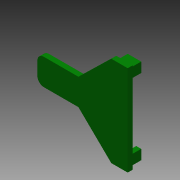
# Autodesk Inventor part: Front Sensor Holder
Saved by Autodesk Inventor 2014 (Build 180170000, 170)
## iProperties
Created: 2016-02-03
Part Number: Front Sensor Holder
Material: Generic
Document SubType Name: Modeling
Designer: Paul
Density: 1 g/cm^3
Appearance: Dark Green
Author: Paul
Autodesk Inventor part; units mm, degrees
ref_plane "YZ Plane" through (0, 0, 0) normal (1, 0, 0) x (0, 1, 0)
ref_plane "XZ Plane" through (0, 0, 0) normal (0, 1, 0) x (-1, 0, 0)
ref_plane "XY Plane" through (0, 0, 0) normal (0, 0, 1) x (1, 0, 0)
sketch "Sketch1" plane through (0, 0, 0) normal (0, 1, 0) x (-1, 0, 0)
  line L0 (6, 8) -> (-15, 8)
  line L1 (-15, -8) -> (6, -8)
  line L2 (10, -4) -> (10, 4)
  line L3 (-45, 0) -> (10, 0) construction
  arc A0 (10, 4) -> (6, 8) centre (6, 4) ccw
  arc A1 (6, -8) -> (10, -4) centre (6, -4) ccw
  line L4 (-35, 27.5) -> (-15, 8)
  line L5 (-15, -8) -> (-35, -27.5)
  line L6 (-35, 27.5) -> (-45, 27.5)
  line L7 (-45, 27.5) -> (-45, -27.5)
  line L8 (-45, -27.5) -> (-35, -27.5)
  point P0 (0, 0)
  point P1 (10, 8)
  point P2 (10, -8)
  dimension "d1" = 16
  dimension "d3" = 10
  dimension "d4" = 4
  dimension "d16" = 20
  dimension "d17" = 10
  dimension "d18" = 55
  dimension "d26" = 25
  constraints: 18 end point, 5 point on line, 4 point on circle, 4 tangent, 3 parallel, 2 centre point, 2 midpoint, 2 vertical, 1 equal length, 1 equal radius, 1 horizontal, 1 perpendicular, 1 other
  measures "d1" distance of point (10, -8) point (10, 8)
  measures "d3" distance from line of point (0, 0) L2
  measures "d4" radius of A0
  measures "d16" horizontal distance of L4.start L0.end
  measures "d17" distance of L4.start L6.end
  measures "d18" distance of L6.end L7.end
  measures "d26" distance from line of L0.end L2
extrude "Extrusion1" add sketch "Sketch1" along normal blind 3.1
sketch "Sketch2" plane through (0, 3.1, 0) normal (0, 1, 0) x (1, 0, 0)
  line L0 (-7.3, -4.8) -> (7.3, -4.8)
  line L1 (7.3, -4.8) -> (7.3, 4.8)
  line L2 (7.3, 4.8) -> (-7.3, 4.8)
  line L3 (-7.3, 4.8) -> (-7.3, -4.8)
  line L4 (-7.3, -4.8) -> (7.3, 4.8) construction
  line L5 (7.3, -4.8) -> (-7.3, 4.8) construction
  point P0 (0, 0)
  dimension "d7" = 15
  dimension "d8" = 10
  constraints: 12 end point, 2 midpoint, 2 parallel, 1 horizontal, 1 perpendicular
extrude "Extrusion2" add sketch "Sketch2" along normal blind 1.5
fillet "Fillet1" radius 2 4 edges at (7.3, 3.85, -4.8) (7.3, 3.85, 4.8) (-7.3, 3.85, 4.8) (-7.3, 3.85, -4.8)
sketch "Sketch3" plane through (0, 3.1, 0) normal (0, 1, 0) x (1, 0, 0)
  line L0 (-10, 4) -> (-10, -4) projected
  line L1 (35, -27.5) -> (45, -27.5) projected
  line L2 (45, -27.5) -> (45, 27.5) projected
  line L3 (15, 8) -> (-6, 8) projected
  line L4 (35.9, 20) -> (38.9, 20)
  line L5 (38.9, 20) -> (38.9, 23)
  line L6 (38.9, 23) -> (41.1, 23)
  line L7 (41.1, 23) -> (41.1, 20)
  line L8 (41.1, 20) -> (44.1, 20)
  line L9 (44.1, 20) -> (44.1, 26)
  line L10 (44.1, 26) -> (35.9, 26)
  line L11 (35.9, 26) -> (35.9, 20)
  line L12 (45, 0) -> (-10, 0) construction
  line L13 (35.9, -20) -> (38.9, -20)
  line L14 (38.9, -20) -> (38.9, -23)
  line L15 (38.9, -23) -> (41.1, -23)
  line L16 (41.1, -23) -> (41.1, -20)
  line L17 (41.1, -20) -> (44.1, -20)
  line L18 (44.1, -20) -> (44.1, -26)
  line L19 (44.1, -26) -> (35.9, -26)
  line L20 (35.9, -26) -> (35.9, -20)
  line L21 (35, 27.5) -> (35, -27.5) construction
  line L22 (45, 27.5) -> (35, 27.5) projected
  line L23 (40, -27.5) -> (40, 27.5) construction
  point P0 (0, 0)
  point P1 (40, 26)
  dimension "d19" = 3
  dimension "d20" = 3
  dimension "d21" = 1.6
  dimension "d22" = 45.4
  constraints: 38 end point, 12 parallel, 9 equal length, 5 midpoint, 3 perpendicular, 2 collinear, 1 point on line, 1 vertical alignment, 1 other
  measures "d19" distance between parallel lines of L10 L6
  measures "d20" distance of L4.start L4.end
extrude "Extrusion3" add sketch "Sketch3" along normal blind 6
equation "\"d20\" = d19"
body "Solid1"
